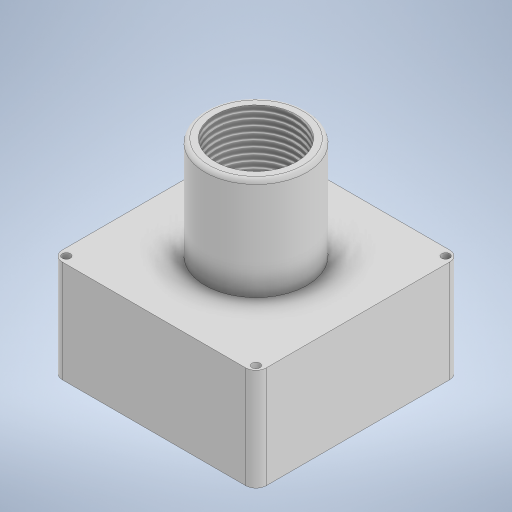
# Autodesk Inventor part: Part1
Saved by Autodesk Inventor 2024 (Build 280153000, 153)
## iProperties
Created: 2024-02-13
Part Number: Part1
Material: Generic
Document SubType Name: Modeling
Designer: Jorge morales
Density: 1 g/cm^3
Appearance: Default
Author: Jorge morales
Autodesk Inventor part; units mm, degrees
ref_plane "YZ Plane" through (0, 0, 0) normal (1, 0, 0) x (0, 1, 0)
ref_plane "XZ Plane" through (0, 0, 0) normal (0, 1, 0) x (-1, 0, 0)
ref_plane "XY Plane" through (0, 0, 0) normal (0, 0, 1) x (1, 0, 0)
sketch "Sketch1" plane through (0, 0, 0) normal (0, 1, 0) x (-1, 0, 0)
  line L0 (-50, 45) -> (-50, -45)
  line L1 (-45, -50) -> (45, -50)
  line L2 (50, -45) -> (50, 45)
  line L3 (45, 50) -> (-45, 50)
  circle A0 centre (46.4645, 46.4645) radius 2
  arc A1 (50, 45) -> (45, 50) centre (45, 45) ccw
  circle A2 centre (45.0503, -45.0503) radius 2
  arc A3 (45, -50) -> (50, -45) centre (45, -45) ccw
  line L4 (48.5355, -48.5355) -> (50, -50) construction
  circle A4 centre (-46.4645, 46.4645) radius 2
  circle A5 centre (-46.4645, -46.4645) radius 2
  arc A6 (-45, 50) -> (-50, 45) centre (-45, 45) ccw
  arc A7 (-50, -45) -> (-45, -50) centre (-45, -45) ccw
  line L5 (-50, 50) -> (-47.8787, 47.8787) construction
  line L6 (-45.0503, 45.0503) -> (46.4645, -46.4645) construction
  line L7 (-50, -50) -> (-47.8787, -47.8787) construction
  line L8 (-45.0503, -45.0503) -> (45.0503, 45.0503) construction
  point P0 (0, 0)
  dimension "d0" = 100
  dimension "d1" = 100
  constraints: 18 end point, 13 point on circle, 8 tangent, 7 point on line, 6 centre point, 2 parallel, 1 equal radius, 1 midpoint, 1 perpendicular, 1 vertical, 6 other
  measures "d0" distance of L5.start L7.start
  measures "d1" distance of L4.end L7.start
extrude "Extrusion1" add sketch "Sketch1" along normal blind 50
sketch "Sketch2" plane through (0, 50, 0) normal (0, 1, 0) x (1, 0, 0)
  circle A0 centre (0, 0) radius 25
  constraints: 1 centre point, 1 coincident
extrude "Extrusion2" add sketch "Sketch2" along normal blind 50
sketch "Sketch3" plane through (0, 100, 0) normal (0, 1, 0) x (1, 0, 0)
  circle A0 centre (0, 0) radius 20
  dimension "d18" = 40
  constraints: 1 centre point, 1 coincident
  measures "d18" diameter of A0
extrude "Extrusion3" cut sketch "Sketch3" against normal blind 30
thread "Thread1" size "M40x3" class "6H" standard "ANSI Metric M Profile" full length
fillet "Fillet1" radius 2 1 edges at (-25, 100, 0)
body "Solid1"
